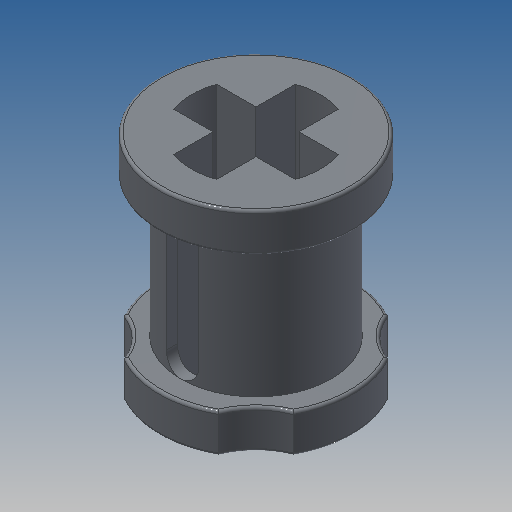
# Autodesk Inventor part: 3713-LtBluishGray
Saved by Autodesk Inventor 2022.2 (Build 262287000, 287)
## iProperties
Created: 2012-10-28
Part Number: 3713-LtBluishGray
Material: ABS Plastic
Document SubType Name: Modeling
Designer: D. Kohfeld
Mass: 0.143934 g
Surface Area: 3.68274 cm^2
Volume: 0.135787 cm^3
Density: 1.06 g/cm^3
Appearance: LtBluishGray
Author: D. Kohfeld
Autodesk Inventor part; units mm, degrees
ref_plane "YZ Plane" through (0, 0, 0) normal (1, 0, 0) x (0, 1, 0)
ref_plane "XZ Plane" through (0, 0, 0) normal (0, 1, 0) x (-1, 0, 0)
ref_plane "XY Plane" through (0, 0, 0) normal (0, 0, 1) x (1, 0, 0)
sketch "Sketch10" plane through (0, 0, 0) normal (0, 1, 0) x (-1, 0, 0)
  circle A0 centre (0, 0) radius 2.8
  dimension "d65" = 5.6
  constraints: 1 centre point, 1 coincident
  measures "d65" diameter of A0
extrude "Extrusion20" add sketch "Sketch10" along normal mid plane 8
sketch "Sketch11" plane through (0, -4, 0) normal (0, -1, 0) x (1, 0, 0)
  circle A0 centre (0, 0) radius 3.6
  circle A1 centre (0, 0) radius 2.8 projected
  point P0 (-7.7315, 0)
  dimension "d69" = 7.2
  constraints: 1 centre point, 1 coincident
  measures "d69" diameter of A0
extrude "Extrusion21" add sketch "Sketch11" against normal blind 1.44
mirror "Mirror4" about plane through (0, 0, 0) normal (0, 1, 0) of "Extrusion21"
sketch "Sketch14" plane through (0, -4, 0) normal (0, -1, 0) x (1, 0, 0)
  arc A0 (-2.2627, 0.8) -> (-2.2627, -0.8) centre (0, 0) ccw
  line L0 (-2.2627, 0.8) -> (-0.8, 0.8)
  line L1 (2.2627, -0.8) -> (0.8, -0.8)
  line L2 (0.8, 2.2627) -> (0.8, 0.8)
  line L3 (-0.8, -2.2627) -> (-0.8, -0.8)
  line L4 (0.8, 0.8) -> (0.8, -0.8) construction
  line L5 (0.8, -0.8) -> (0.8, -2.2627)
  line L6 (0.8, -0.8) -> (-0.8, -0.8) construction
  line L7 (-0.8, -0.8) -> (-2.2627, -0.8)
  line L8 (-0.8, -0.8) -> (-0.8, 0.8) construction
  line L9 (-0.8, 0.8) -> (-0.8, 2.2627)
  line L10 (0.8, 0.8) -> (2.2627, 0.8)
  line L11 (-0.8, 0.8) -> (0.8, 0.8) construction
  arc A1 (-0.8, 2.2627) -> (-2.2627, 0.8) centre (0, 0) ccw construction
  arc A2 (2.2627, 0.8) -> (0.8, 2.2627) centre (0, 0) ccw construction
  arc A3 (0.8, 2.2627) -> (-0.8, 2.2627) centre (0, 0) ccw
  arc A4 (2.2627, -0.8) -> (2.2627, 0.8) centre (0, 0) ccw
  arc A5 (0.8, -2.2627) -> (2.2627, -0.8) centre (0, 0) ccw construction
  arc A6 (-0.8, -2.2627) -> (0.8, -2.2627) centre (0, 0) ccw
  arc A7 (-2.2627, -0.8) -> (-0.8, -2.2627) centre (0, 0) ccw construction
  circle A8 centre (0, 0) radius 3.6 projected
  point P0 (-8, 0)
  point P1 (0.8, 0)
  point P2 (0, -0.8)
  dimension "d81" = 4.8
  dimension "d82" = 1.6
  dimension "d83" = 1.6
  constraints: 27 point on circle, 24 end point, 18 parallel, 8 centre point, 3 horizontal, 2 midpoint, 1 coincident, 1 horizontal alignment, 1 vertical, 1 vertical alignment
  measures "d81" diameter of A0
  measures "d82" distance between parallel lines of L2 L3
  measures "d83" distance between parallel lines of L1 L0
extrude "Extrusion23" cut sketch "Sketch14" against normal through all contours L0 L9 A3 L2 L10 A4 L1 L5 A6 L3 L7 A0
sketch "Sketch16" plane through (0, 0, 0) normal (0, 0, 1) x (1, 0, 0)
  line L0 (0.6, 1.96) -> (0.6, -1.96)
  line L1 (-0.6, -1.96) -> (-0.6, 1.96)
  arc A0 (0.6, 1.96) -> (-0.6, 1.96) centre (0, 1.96) ccw
  arc A1 (-0.6, -1.96) -> (0.6, -1.96) centre (0, -1.96) ccw
  line L2 (-0.8, 4) -> (0.8, 4) projected
  line L3 (2.2627, 4) -> (2.2627, 4) projected
  line L4 (2.8, -2.56) -> (2.8, 2.56) projected
  line L5 (3.6, 2.56) -> (3.6, 2.56) projected
  point P0 (0.6, 0)
  point P1 (2.8, 0)
  point P2 (0, 4)
  dimension "d99" = 1.2
  constraints: 5 tangent, 4 end point, 4 point on circle, 3 midpoint, 2 centre point, 1 coincident, 1 horizontal alignment, 1 parallel, 1 vertical, 1 vertical alignment
  measures "d99" diameter of A0
extrude "Extrusion24" cut sketch "Sketch16" along normal through all both and the other way through all
sketch "Sketch22" plane through (0, -4, 0) normal (0, -1, 0) x (1, 0, 0)
  arc A0 (-2.2627, 0.8) -> (-2.2627, -0.8) centre (0, 0) ccw projected
  line L0 (-0.8, -0.8) -> (-2.2627, -0.8) projected
  circle A1 centre (-4, 4) radius 2.4
  circle A2 centre (4, 4) radius 2.4
  circle A3 centre (-4, -4) radius 2.4
  circle A4 centre (4, -4) radius 2.4
  line L1 (-4, -4) -> (-4, 4) construction
  line L2 (-4, 4) -> (4, 4) construction
  point P0 (0, 4)
  point P1 (-4, 0)
  dimension "d142" = 8
  dimension "d143" = 4.8
  constraints: 4 centre point, 4 end point, 3 equal radius, 3 perpendicular, 2 horizontal alignment, 2 midpoint, 2 vertical alignment
  measures "d142" distance of L1.end L2.end
  measures "d143" diameter of A1
extrude "Extrusion29" cut sketch "Sketch22" against normal up to surface (1.44 mm away)
fillet "Fillet7" radius 0.1 18 edges at (3.6, -4, 0) (0, -4, 3.6) (-3.6, -4, 0) (0, -4, -3.6) (-2.3029, -4, 2.3029) (-2.3029, -4, -2.3029) (2.3029, -4, -2.3029) (2.3029, -4, 2.3029) (2.3029, -2.56, 2.3029) (3.6, -2.56, 0) (-3.6, 2.56, 0) (-3.6, 4, 0) (0, -2.56, 3.6) (-2.3029, -2.56, 2.3029) (-3.6, -2.56, 0) (-2.3029, -2.56, -2.3029) (0, -2.56, -3.6) (2.3029, -2.56, -2.3029)
body "Solid1"
body "Solid2"
